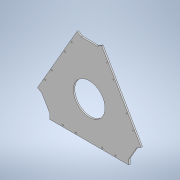
# Autodesk Inventor part: HexChris
Saved by Autodesk Inventor 2020 (Build 240168000, 168)
## iProperties
Created: 2020-03-20
Part Number: HexChris
Material: Generic
Document SubType Name: Modeling
Designer: srini
Density: 1 g/cm^3
Appearance: Default
Author: srini
Autodesk Inventor part; units mm, degrees
ref_plane "YZ Plane" through (0, 0, 0) normal (1, 0, 0) x (0, 1, 0)
ref_plane "XZ Plane" through (0, 0, 0) normal (0, 1, 0) x (-1, 0, 0)
ref_plane "XY Plane" through (0, 0, 0) normal (0, 0, 1) x (1, 0, 0)
sketch "Sketch1" plane through (0, 0, 0) normal (0, 0, 1) x (1, 0, 0)
  circle A0 centre (0, 300.2176) radius 127
  circle A1 centre (-352.7667, 256.8867) radius 4
  circle A2 centre (-299.8517, 348.5382) radius 4
  circle A3 centre (-194.0217, 531.8411) radius 4
  circle A4 centre (-141.1067, 623.4926) radius 4
  circle A5 centre (141.0967, 623.5099) radius 4
  circle A6 centre (194.0117, 531.8584) radius 4
  circle A7 centre (299.8417, 348.5555) radius 4
  circle A8 centre (352.7567, 256.904) radius 4
  circle A9 centre (211.67, 12.5) radius 4
  circle A10 centre (105.84, 12.5) radius 4
  circle A11 centre (-105.82, 12.5) radius 4
  circle A12 centre (-211.65, 12.5) radius 4
  line L0 (0, 0) -> (317.5, 0)
  line L1 (0, 0) -> (-315.5021, 0)
  line L2 (-315.5021, 0) -> (-315.5021, 41)
  line L3 (317.5, 0) -> (317.5, 41)
  line L4 (-315.5021, 41) -> (-379.0021, 150.9852)
  line L5 (-379.0021, 150.9852) -> (-414.5086, 171.4861)
  line L6 (-414.5086, 171.4861) -> (-98.007, 719.6793)
  line L7 (-98.007, 719.6793) -> (-62.5, 699.1793)
  line L8 (-62.5, 699.1793) -> (64.5, 699.1793)
  line L9 (64.5, 699.1793) -> (100.007, 719.6793)
  line L10 (100.007, 719.6793) -> (416.507, 171.4852)
  line L11 (416.507, 171.4852) -> (381, 150.9852)
  line L12 (381, 150.9852) -> (317.5, 41)
  line L13 (-414.5086, 171.4861) -> (-402.1778, 164.3665)
  line L14 (100.007, 719.6793) -> (90.601, 714.2488)
  line L15 (-315.5021, 0) -> (-315.5021, 12.5)
  point P0 (0, 297.6322)
  point P1 (317.5, 41)
  constraints: 32 end point, 13 centre point
extrude "Extrusion1" add sketch "Sketch1" along normal blind 11.1125
body "Solid1"
